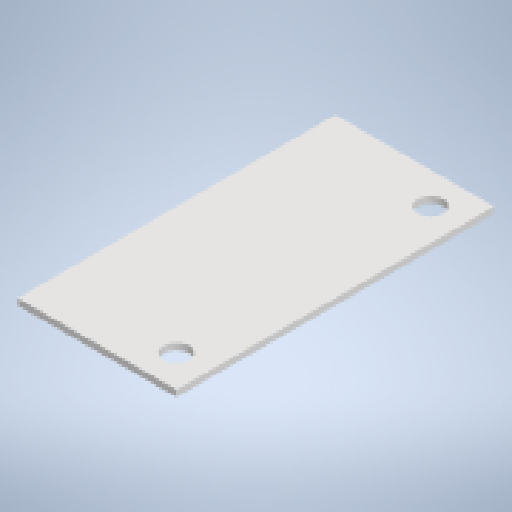
# Autodesk Inventor part: H
Saved by Autodesk Inventor 2023 (Build 270158000, 158)
## iProperties
Created: 2022-11-06
Part Number: H
Material: Generic
Document SubType Name: Modeling
Designer: SAMJ
Density: 1 g/cm^3
Appearance: Default
Author: SAMJ
Autodesk Inventor part; units mm, degrees
ref_plane "YZ Plane" through (0, 0, 0) normal (1, 0, 0) x (0, 1, 0)
ref_plane "XZ Plane" through (0, 0, 0) normal (0, 1, 0) x (-1, 0, 0)
ref_plane "XY Plane" through (0, 0, 0) normal (0, 0, 1) x (1, 0, 0)
sketch "Sketch1" plane through (0, 0, 0) normal (0, 1, 0) x (-1, 0, 0)
  line L0 (-25, 50) -> (25, 50)
  line L1 (25, 50) -> (25, -50)
  line L2 (25, -50) -> (-25, -50)
  line L3 (-25, -50) -> (-25, 50)
  line L4 (-25, 50) -> (25, -50) construction
  line L5 (25, 50) -> (-25, -50) construction
  line L6 (-25, 50) -> (-25, 40)
  line L7 (-25, 40) -> (-15, 40)
  circle A0 centre (-15, 40) radius 4
  line L8 (-25, -50) -> (-25, -40)
  line L9 (-25, -40) -> (-15, -40)
  circle A1 centre (-15, -40) radius 4
  point P0 (0, 0)
  dimension "d0" = 50
  dimension "d1" = 100
  dimension "d8" = 10
  dimension "d9" = 10
  dimension "d10" = 8
  dimension "d11" = 10
  dimension "d12" = 10
  dimension "d13" = 8
  constraints: 20 end point, 3 perpendicular, 2 centre point, 2 coincident, 2 midpoint, 2 parallel, 2 point on line, 1 horizontal
  measures "d0" distance of L1.end L2.end
  measures "d1" distance of L0.end L1.end
  measures "d8" distance of L0.start L6.end
  measures "d9" distance of L6.end L7.end
  measures "d10" diameter of A0
  measures "d11" distance of L2.end L8.end
  measures "d12" distance of L8.end L9.end
  measures "d13" diameter of A1
extrude "Extrusion2" add sketch "Sketch1" along normal blind 2
body "Solid2"
